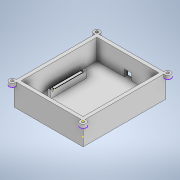
# Autodesk Inventor part: Spod
Saved by Autodesk Inventor 2021 (Build 250183000, 183)
## iProperties
Created: 2021-01-03
Part Number: Spod
Material: Generic
Document SubType Name: Modeling
Designer: emili
Density: 1 g/cm^3
Appearance: Default
Author: emili
Autodesk Inventor part; units mm, degrees
ref_plane "YZ Plane" through (0, 0, 0) normal (1, 0, 0) x (0, 1, 0)
ref_plane "XZ Plane" through (0, 0, 0) normal (0, 1, 0) x (-1, 0, 0)
ref_plane "XY Plane" through (0, 0, 0) normal (0, 0, 1) x (1, 0, 0)
sketch "Sketch2" plane through (0, 0, 0) normal (0, 1, 0) x (-1, 0, 0)
  line L0 (0, 0) -> (100, 0)
  line L1 (100, 0) -> (100, -120)
  line L2 (100, -120) -> (0, -120)
  line L3 (0, -120) -> (0, 0)
  dimension "d0" = 100
  dimension "d1" = 120
  constraints: 8 end point, 2 parallel, 1 horizontal, 1 perpendicular
  measures "d0" distance of L1.end L2.end
  measures "d1" distance of L0.end L1.end
extrude "Extrusion1" add sketch "Sketch2" along normal blind 3
sketch "Sketch3" plane through (0, 3, 0) normal (0, 1, 0) x (1, 0, 0)
  line L0 (0, 120) -> (-100, 120) projected
  line L1 (-100, 120) -> (-100, 0) projected
  line L2 (-95, 115) -> (-5, 115)
  line L3 (-5, 115) -> (-5, 5)
  line L4 (-5, 5) -> (-95, 5)
  line L5 (-95, 5) -> (-95, 115)
  line L6 (-100, 120) -> (0, 120)
  line L7 (0, 120) -> (0, 0)
  line L8 (0, 0) -> (-100, 0)
  line L9 (-100, 0) -> (-100, 120)
  dimension "d6" = 90
  dimension "d7" = 110
  constraints: 16 end point, 4 parallel, 2 horizontal, 2 perpendicular
  measures "d6" distance of L3.end L4.end
  measures "d7" distance of L2.end L3.end
extrude "Extrusion2" add sketch "Sketch3" along normal blind 30
sketch "Sketch4" plane through (0, 3, 0) normal (0, 1, 0) x (1, 0, 0)
  line L0 (-95, 115) -> (-95, 5) projected
  line L1 (-95, 115) -> (-95, 85)
  line L2 (-85, 85) -> (-15, 85)
  line L3 (-15, 85) -> (-15, 35)
  line L4 (-15, 35) -> (-85, 35)
  line L5 (-85, 35) -> (-85, 85)
  line L6 (-85, 85) -> (-81, 85)
  line L7 (-81, 85) -> (-81, 35)
  line L8 (-81, 35) -> (-85, 35)
  line L9 (-85, 35) -> (-85, 85)
  line L10 (-15, 85) -> (-19, 85)
  line L11 (-19, 85) -> (-19, 35)
  line L12 (-19, 35) -> (-15, 35)
  line L13 (-15, 35) -> (-15, 85)
  line L14 (-85, 85) -> (-81, 85)
  line L15 (-81, 85) -> (-81, 81)
  line L16 (-81, 81) -> (-85, 81)
  line L17 (-85, 81) -> (-85, 85)
  line L18 (-85, 35) -> (-81, 35)
  line L19 (-81, 35) -> (-81, 39)
  line L20 (-81, 39) -> (-85, 39)
  line L21 (-85, 39) -> (-85, 35)
  line L22 (-19, 35) -> (-15, 35)
  line L23 (-15, 35) -> (-15, 39)
  line L24 (-15, 39) -> (-19, 39)
  line L25 (-19, 39) -> (-19, 35)
  line L26 (-19, 85) -> (-15, 85)
  line L27 (-15, 85) -> (-15, 81)
  line L28 (-15, 81) -> (-19, 81)
  line L29 (-19, 81) -> (-19, 85)
  circle A0 centre (-83, 83) radius 1
  circle A1 centre (-83, 37) radius 1
  circle A2 centre (-17, 37) radius 1
  circle A3 centre (-17, 83) radius 1
  point P0 (0, 0)
  dimension "d12" = 70
  dimension "d13" = 50
  dimension "d14" = 4
  dimension "d15" = 4
  dimension "d16" = 4
  dimension "d17" = 4
  dimension "d18" = 2
  dimension "d19" = 2
  dimension "d20" = 2
  constraints: 58 end point, 14 parallel, 9 point on line, 7 horizontal, 7 perpendicular, 4 centre point
  measures "d12" distance of L3.end L4.end
  measures "d13" distance of L2.end L3.end
  measures "d14" distance of L7.end L8.end
  measures "d15" distance of L12.end L11.end
  measures "d16" distance of L14.end L15.end
  measures "d17" distance of L19.end L18.end
  measures "d18" diameter of A0
  measures "d19" diameter of A1
  measures "d20" diameter of A2
sketch "Sketch5" plane through (0, 33, 0) normal (0, 1, 0) x (1, 0, 0)
  point P0 (0, 0)
sketch "Sketch6" plane through (0, 33, 0) normal (0, 1, 0) x (1, 0, 0)
  line L0 (-100, 0) -> (0, 0) projected
  line L1 (0, 0) -> (10, 0) construction
  circle A0 centre (1.4142, -1.4142) radius 2
  circle A1 centre (1.4142, -1.4142) radius 4.5
  circle A2 centre (1.4084, 121.4127) radius 2
  circle A3 centre (1.4084, 121.4127) radius 4.5
  circle A4 centre (-101.4585, 121.4298) radius 2
  circle A5 centre (-101.4585, 121.4298) radius 4.5
  circle A6 centre (-101.4195, -1.4184) radius 2
  circle A7 centre (-101.4195, -1.4184) radius 4.5
  dimension "d24" = 4
  dimension "d25" = 9
  dimension "d27" = 4
  dimension "d28" = 9
  dimension "d30" = 4
  dimension "d31" = 9
  dimension "d33" = 4
  dimension "d34" = 9
  constraints: 8 centre point, 4 coincident, 2 end point, 1 horizontal
  measures "d24" diameter of A0
  measures "d25" diameter of A1
  measures "d27" diameter of A2
  measures "d28" diameter of A3
  measures "d30" diameter of A4
  measures "d31" diameter of A5
  measures "d33" diameter of A6
  measures "d34" diameter of A7
extrude "Extrusion3" add sketch "Sketch6" against normal blind 5
extrude "Extrusion4" add sketch "Sketch4" along normal blind 10 contours L16 L7 L20 L5 | L28 L3 L24 L11
sketch "Sketch7" plane through (0, 13, 0) normal (0, 1, 0) x (1, 0, 0)
  point P0 (0, 0)
sketch "Sketch10" plane through (0, 13, 0) normal (0, 1, 0) x (1, 0, 0)
  line L0 (-81, 81) -> (-85, 81) projected
  line L1 (-81, 39) -> (-81, 81) projected
  line L2 (-85, 81) -> (-81, 81)
  line L3 (-81, 81) -> (-81, 39)
  line L4 (-81, 39) -> (-85, 39)
  line L5 (-85, 39) -> (-85, 81)
  point P0 (0, 0)
  constraints: 8 end point, 2 parallel, 1 horizontal, 1 perpendicular
sketch "Sketch11" plane through (0, 13, 0) normal (0, 1, 0) x (1, 0, 0)
  line L0 (-15, 81) -> (-19, 81) projected
  line L1 (-15, 39) -> (-15, 81) projected
  line L2 (-19, 81) -> (-15, 81)
  line L3 (-15, 81) -> (-15, 39)
  line L4 (-15, 39) -> (-19, 39)
  line L5 (-19, 39) -> (-19, 81)
  line L6 (-85, 81) -> (-81, 81) projected
  line L7 (-85, 81) -> (-81, 81)
  line L8 (-81, 81) -> (-81, 85)
  line L9 (-81, 85) -> (-85, 85)
  line L10 (-85, 85) -> (-85, 81)
  line L11 (-19, 39) -> (-19, 81) projected
  line L12 (-19, 81) -> (-15, 81)
  line L13 (-15, 81) -> (-15, 85)
  line L14 (-15, 85) -> (-19, 85)
  line L15 (-19, 85) -> (-19, 81)
  line L16 (-15, 39) -> (-19, 39) projected
  line L17 (-19, 39) -> (-15, 39)
  line L18 (-15, 39) -> (-15, 35)
  line L19 (-15, 35) -> (-19, 35)
  line L20 (-19, 35) -> (-19, 39)
  line L21 (-85, 39) -> (-81, 39)
  line L22 (-81, 39) -> (-81, 35)
  line L23 (-81, 35) -> (-85, 35)
  line L24 (-85, 35) -> (-85, 39)
  circle A0 centre (-83, 83) radius 1
  circle A1 centre (-17, 83) radius 1
  circle A2 centre (-17, 37) radius 1
  circle A3 centre (-83, 37) radius 1
  line L25 (-19, 84.1547) -> (-17, 85.3094)
  line L26 (-17, 85.3094) -> (-15, 84.1547)
  line L27 (-15, 84.1547) -> (-15, 81.8453)
  line L28 (-15, 81.8453) -> (-17, 80.6906)
  line L29 (-17, 80.6906) -> (-19, 81.8453)
  line L30 (-19, 81.8453) -> (-19, 84.1547)
  line L31 (-19, 38.1547) -> (-17, 39.3094)
  line L32 (-17, 39.3094) -> (-15, 38.1547)
  line L33 (-15, 38.1547) -> (-15, 35.8453)
  line L34 (-15, 35.8453) -> (-17, 34.6906)
  line L35 (-17, 34.6906) -> (-19, 35.8453)
  line L36 (-19, 35.8453) -> (-19, 38.1547)
  line L37 (-81, 35.8453) -> (-83, 34.6906)
  line L38 (-83, 34.6906) -> (-85, 35.8453)
  line L39 (-85, 35.8453) -> (-85, 38.1547)
  line L40 (-85, 38.1547) -> (-83, 39.3094)
  line L41 (-83, 39.3094) -> (-81, 38.1547)
  line L42 (-81, 38.1547) -> (-81, 35.8453)
  line L43 (-81, 81.8453) -> (-83, 80.6906)
  line L44 (-83, 80.6906) -> (-85, 81.8453)
  line L45 (-85, 81.8453) -> (-85, 84.1547)
  line L46 (-85, 84.1547) -> (-83, 85.3094)
  line L47 (-83, 85.3094) -> (-81, 84.1547)
  line L48 (-81, 84.1547) -> (-81, 81.8453)
  point P0 (0, 0)
  point P1 (-19, 83)
  point P2 (-19, 37)
  point P3 (-81, 37)
  point P4 (-81, 83)
  dimension "d75" = 4
  dimension "d76" = 4
  dimension "d77" = 2
  dimension "d78" = 2
  dimension "d79" = 2
  constraints: 88 end point, 10 parallel, 8 midpoint, 6 point on line, 5 coincident, 5 horizontal, 5 perpendicular, 4 centre point, 52 other
  measures "d75" distance of L8.end L7.end
  measures "d76" distance of L17.end L18.end
  measures "d77" diameter of A0
  measures "d78" diameter of A1
  measures "d79" diameter of A2
sketch "Sketch17" plane through (0, 3, 0) normal (0, 1, 0) x (1, 0, 0)
  line L0 (-85, 85) -> (-15, 85)
  line L1 (-15, 85) -> (-15, 35)
  line L2 (-15, 35) -> (-85, 35)
  line L3 (-85, 35) -> (-85, 85)
  line L4 (-85, 85) -> (-81, 85)
  line L5 (-81, 85) -> (-81, 35)
  line L6 (-81, 35) -> (-85, 35)
  line L7 (-85, 35) -> (-85, 85)
  line L8 (-15, 85) -> (-19, 85)
  line L9 (-19, 85) -> (-19, 35)
  line L10 (-19, 35) -> (-15, 35)
  line L11 (-15, 35) -> (-15, 85)
  point P0 (0, 0)
  point P1 (-95, 115)
  constraints: 24 end point, 6 parallel, 3 horizontal, 3 perpendicular, 2 point on line
extrude "Extrusion7" add sketch "Sketch17" along normal blind 10 contours L0 L5 L2 L3 | L0 L1 L2 L9
sketch "Sketch18" plane through (0, 3, 0) normal (0, 1, 0) x (1, 0, 0)
  line L0 (-19, 35) -> (-19, 85) projected
  line L1 (-19, 35) -> (-15, 35)
  line L2 (-15, 35) -> (-15, 33.5)
  line L3 (-15, 33.5) -> (-19, 33.5)
  line L4 (-19, 33.5) -> (-19, 35)
  line L5 (-19, 85) -> (-15, 85)
  line L6 (-15, 85) -> (-15, 86.5)
  line L7 (-15, 86.5) -> (-19, 86.5)
  line L8 (-19, 86.5) -> (-19, 85)
  line L9 (-81, 85) -> (-85, 85) projected
  line L10 (-85, 85) -> (-81, 85)
  line L11 (-81, 85) -> (-81, 86.5)
  line L12 (-81, 86.5) -> (-85, 86.5)
  line L13 (-85, 86.5) -> (-85, 85)
  line L14 (-85, 35) -> (-81, 35) projected
  line L15 (-85, 35) -> (-81, 35)
  line L16 (-81, 35) -> (-81, 33.5)
  line L17 (-81, 33.5) -> (-85, 33.5)
  line L18 (-85, 33.5) -> (-85, 35)
  point P0 (0, 0)
  dimension "d80" = 4
  dimension "d81" = 1.5
  dimension "d82" = 1.5
  constraints: 32 end point, 8 parallel, 4 horizontal, 4 perpendicular, 4 point on line
  measures "d80" distance of L2.end L3.end
  measures "d81" distance of L1.end L2.end
  measures "d82" distance of L6.end L5.end
extrude "Extrusion8" add sketch "Sketch18" along normal blind 10
extrude "Extrusion9" cut sketch "Sketch11" against normal blind 2 contours L28 L29 L0 | L0 L29 L15 L25 L14 L26 L13 L28 | L32 L18 L34 L19 L35 L20 L31 L4 | L4 L31 L32 | L14 L25 L26 | L34 L35 L19 | L44 L10 L46 L9 L47 L8 L43 L6 | L6 L43 L44 | L46 L47 L9 | L40 L41 L21 | L21 L41 L22 L37 L23 L38 L24 L40 | L23 L37 L38 | A0 | A1 | A2 | A3
sketch "Sketch19" plane through (0, 28, 0) normal (0, -1, 0) x (1, 0, 0)
  circle A0 centre (1.4142, 1.4142) radius 2 projected
  circle A1 centre (1.4142, 1.4142) radius 2
  circle A2 centre (1.4142, 1.4142) radius 4.5
  circle A3 centre (-101.4195, 1.4184) radius 2 projected
  circle A4 centre (-101.4195, 1.4184) radius 2
  circle A5 centre (-101.4195, 1.4184) radius 4.5
  circle A6 centre (-101.4585, -121.4298) radius 2 projected
  circle A7 centre (-101.4585, -121.4298) radius 2
  circle A8 centre (-101.4585, -121.4298) radius 4.5
  circle A9 centre (1.4142, -121.4298) radius 2.0171
  arc A10 (-0.0073, -120) -> (0, -119.9927) centre (1.4084, -121.4127) ccw projected
  circle A11 centre (1.4084, -121.4127) radius 4.5
  point P0 (0, 0)
  constraints: 8 centre point, 7 coincident, 1 other
sketch "Sketch20" plane through (0, 0, -120) normal (0, 0, -1) x (-1, 0, 0)
  line L0 (100, 28) -> (100, 33) projected
  line L1 (0, 0) -> (100, 0)
  line L2 (100, 0) -> (100, 33)
  line L3 (100, 33) -> (0, 33)
  line L4 (0, 33) -> (0, 0)
  line L5 (95, 3) -> (5, 3) projected
  line L6 (50, 3) -> (55, 3)
  line L7 (55, 3) -> (55, 13)
  line L8 (55, 13) -> (50, 13)
  line L9 (50, 13) -> (45, 13)
  line L10 (45, 13) -> (45, 3)
  line L11 (45, 3) -> (50, 3)
  line L12 (55, 13) -> (45, 13)
  line L13 (45, 13) -> (45, 3)
  line L14 (45, 3) -> (55, 3)
  line L15 (55, 3) -> (55, 13)
  constraints: 28 end point, 6 parallel, 4 horizontal, 4 perpendicular, 1 midpoint, 1 point on line
extrude "Extrusion10" cut sketch "Sketch20" against normal blind 10 contours L5 L10 L9 L8 L7
body "Solid1"
